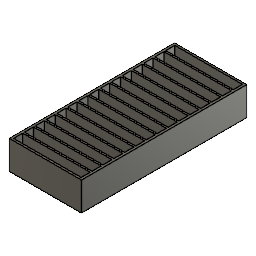
GBA Stand v4 (Autodesk Fusion 360 design; units mm, degrees)
Autodesk Fusion 360 part; units mm, degrees
sketch "Sketch1" plane through (0, 0, 0) normal (0, 1, 0) x (1, 0, 0)
  line L0 (2.75, 1.25) -> (2.75, 0)
  line L1 (2.75, 1.25) -> (54.15, 1.25)
  line L2 (54.15, 1.25) -> (54.15, 5.25)
  line L3 (54.15, 5.25) -> (2.75, 5.25)
  line L4 (2.75, 5.25) -> (2.75, 1.25)
  line L5 (0, 0) -> (56.9, 0)
  line L6 (56.9, 0) -> (56.9, 7.3)
  line L7 (56.9, 7.3) -> (0, 7.3)
  line L8 (0, 7.3) -> (0, 0)
  line L9 (-2, -2) -> (58.9, -2)
  line L10 (58.9, -2) -> (58.9, 9.3)
  line L11 (58.9, 9.3) -> (-2, 9.3)
  line L12 (-2, 9.3) -> (-2, -2)
  line L13 (58.9, -2) -> (58.9, 9.3)
  line L14 (58.9, 9.3) -> (-2, 9.3)
  line L15 (-2, 9.3) -> (-2, -2)
  line L16 (-2, -2) -> (58.9, -2)
  line L17 (2.75, 1.25) -> (54.15, 1.25)
  line L18 (2.75, 1.25) -> (2.75, 0)
  line L19 (54.15, 1.25) -> (54.15, 5.25)
  line L20 (54.15, 5.25) -> (2.75, 5.25)
  line L21 (2.75, 5.25) -> (2.75, 1.25)
  line L22 (0, 0) -> (56.9, 0)
  line L23 (56.9, 0) -> (56.9, 7.3)
  line L24 (0, 7.3) -> (0, 0)
  line L25 (56.9, 7.3) -> (0, 7.3)
  line L26 (58.9, 7.3) -> (58.9, 18.6)
  line L27 (58.9, 18.6) -> (-2, 18.6)
  line L28 (-2, 18.6) -> (-2, 7.3)
  line L29 (-2, 7.3) -> (58.9, 7.3)
  line L30 (2.75, 10.55) -> (54.15, 10.55)
  line L31 (2.75, 10.55) -> (2.75, 9.3)
  line L32 (54.15, 10.55) -> (54.15, 14.55)
  line L33 (54.15, 14.55) -> (2.75, 14.55)
  line L34 (2.75, 14.55) -> (2.75, 10.55)
  line L35 (0, 9.3) -> (56.9, 9.3)
  line L36 (56.9, 9.3) -> (56.9, 16.6)
  line L37 (0, 16.6) -> (0, 9.3)
  line L38 (56.9, 16.6) -> (0, 16.6)
  line L39 (58.9, 16.6) -> (58.9, 27.9)
  line L40 (58.9, 27.9) -> (-2, 27.9)
  line L41 (-2, 27.9) -> (-2, 16.6)
  line L42 (-2, 16.6) -> (58.9, 16.6)
  line L43 (2.75, 19.85) -> (54.15, 19.85)
  line L44 (2.75, 19.85) -> (2.75, 18.6)
  line L45 (54.15, 19.85) -> (54.15, 23.85)
  line L46 (54.15, 23.85) -> (2.75, 23.85)
  line L47 (2.75, 23.85) -> (2.75, 19.85)
  line L48 (0, 18.6) -> (56.9, 18.6)
  line L49 (56.9, 18.6) -> (56.9, 25.9)
  line L50 (0, 25.9) -> (0, 18.6)
  line L51 (56.9, 25.9) -> (0, 25.9)
  line L52 (58.9, 25.9) -> (58.9, 37.2)
  line L53 (58.9, 37.2) -> (-2, 37.2)
  line L54 (-2, 37.2) -> (-2, 25.9)
  line L55 (-2, 25.9) -> (58.9, 25.9)
  line L56 (2.75, 29.15) -> (54.15, 29.15)
  line L57 (2.75, 29.15) -> (2.75, 27.9)
  line L58 (54.15, 29.15) -> (54.15, 33.15)
  line L59 (54.15, 33.15) -> (2.75, 33.15)
  line L60 (2.75, 33.15) -> (2.75, 29.15)
  line L61 (0, 27.9) -> (56.9, 27.9)
  line L62 (56.9, 27.9) -> (56.9, 35.2)
  line L63 (0, 35.2) -> (0, 27.9)
  line L64 (56.9, 35.2) -> (0, 35.2)
  line L65 (58.9, 35.2) -> (58.9, 46.5)
  line L66 (58.9, 46.5) -> (-2, 46.5)
  line L67 (-2, 46.5) -> (-2, 35.2)
  line L68 (-2, 35.2) -> (58.9, 35.2)
  line L69 (2.75, 38.45) -> (54.15, 38.45)
  line L70 (2.75, 38.45) -> (2.75, 37.2)
  line L71 (54.15, 38.45) -> (54.15, 42.45)
  line L72 (54.15, 42.45) -> (2.75, 42.45)
  line L73 (2.75, 42.45) -> (2.75, 38.45)
  line L74 (0, 37.2) -> (56.9, 37.2)
  line L75 (56.9, 37.2) -> (56.9, 44.5)
  line L76 (0, 44.5) -> (0, 37.2)
  line L77 (56.9, 44.5) -> (0, 44.5)
  line L78 (58.9, 44.5) -> (58.9, 55.8)
  line L79 (58.9, 55.8) -> (-2, 55.8)
  line L80 (-2, 55.8) -> (-2, 44.5)
  line L81 (-2, 44.5) -> (58.9, 44.5)
  line L82 (2.75, 47.75) -> (54.15, 47.75)
  line L83 (2.75, 47.75) -> (2.75, 46.5)
  line L84 (54.15, 47.75) -> (54.15, 51.75)
  line L85 (54.15, 51.75) -> (2.75, 51.75)
  line L86 (2.75, 51.75) -> (2.75, 47.75)
  line L87 (0, 46.5) -> (56.9, 46.5)
  line L88 (56.9, 46.5) -> (56.9, 53.8)
  line L89 (0, 53.8) -> (0, 46.5)
  line L90 (56.9, 53.8) -> (0, 53.8)
  line L91 (58.9, 53.8) -> (58.9, 65.1)
  line L92 (58.9, 65.1) -> (-2, 65.1)
  line L93 (-2, 65.1) -> (-2, 53.8)
  line L94 (-2, 53.8) -> (58.9, 53.8)
  line L95 (2.75, 57.05) -> (54.15, 57.05)
  line L96 (2.75, 57.05) -> (2.75, 55.8)
  line L97 (54.15, 57.05) -> (54.15, 61.05)
  line L98 (54.15, 61.05) -> (2.75, 61.05)
  line L99 (2.75, 61.05) -> (2.75, 57.05)
  line L100 (0, 55.8) -> (56.9, 55.8)
  line L101 (56.9, 55.8) -> (56.9, 63.1)
  line L102 (0, 63.1) -> (0, 55.8)
  line L103 (56.9, 63.1) -> (0, 63.1)
  line L104 (58.9, 63.1) -> (58.9, 74.4)
  line L105 (58.9, 74.4) -> (-2, 74.4)
  line L106 (-2, 74.4) -> (-2, 63.1)
  line L107 (-2, 63.1) -> (58.9, 63.1)
  line L108 (2.75, 66.35) -> (54.15, 66.35)
  line L109 (2.75, 66.35) -> (2.75, 65.1)
  line L110 (54.15, 66.35) -> (54.15, 70.35)
  line L111 (54.15, 70.35) -> (2.75, 70.35)
  line L112 (2.75, 70.35) -> (2.75, 66.35)
  line L113 (0, 65.1) -> (56.9, 65.1)
  line L114 (56.9, 65.1) -> (56.9, 72.4)
  line L115 (0, 72.4) -> (0, 65.1)
  line L116 (56.9, 72.4) -> (0, 72.4)
  line L117 (58.9, 72.4) -> (58.9, 83.7)
  line L118 (58.9, 83.7) -> (-2, 83.7)
  line L119 (-2, 83.7) -> (-2, 72.4)
  line L120 (-2, 72.4) -> (58.9, 72.4)
  line L121 (2.75, 75.65) -> (54.15, 75.65)
  line L122 (2.75, 75.65) -> (2.75, 74.4)
  line L123 (54.15, 75.65) -> (54.15, 79.65)
  line L124 (54.15, 79.65) -> (2.75, 79.65)
  line L125 (2.75, 79.65) -> (2.75, 75.65)
  line L126 (0, 74.4) -> (56.9, 74.4)
  line L127 (56.9, 74.4) -> (56.9, 81.7)
  line L128 (0, 81.7) -> (0, 74.4)
  line L129 (56.9, 81.7) -> (0, 81.7)
  line L130 (58.9, 81.7) -> (58.9, 93)
  line L131 (58.9, 93) -> (-2, 93)
  line L132 (-2, 93) -> (-2, 81.7)
  line L133 (-2, 81.7) -> (58.9, 81.7)
  line L134 (2.75, 84.95) -> (54.15, 84.95)
  line L135 (2.75, 84.95) -> (2.75, 83.7)
  line L136 (54.15, 84.95) -> (54.15, 88.95)
  line L137 (54.15, 88.95) -> (2.75, 88.95)
  line L138 (2.75, 88.95) -> (2.75, 84.95)
  line L139 (0, 83.7) -> (56.9, 83.7)
  line L140 (56.9, 83.7) -> (56.9, 91)
  line L141 (0, 91) -> (0, 83.7)
  line L142 (56.9, 91) -> (0, 91)
  line L143 (58.9, 91) -> (58.9, 102.3)
  line L144 (58.9, 102.3) -> (-2, 102.3)
  line L145 (-2, 102.3) -> (-2, 91)
  line L146 (-2, 91) -> (58.9, 91)
  line L147 (2.75, 94.25) -> (54.15, 94.25)
  line L148 (2.75, 94.25) -> (2.75, 93)
  line L149 (54.15, 94.25) -> (54.15, 98.25)
  line L150 (54.15, 98.25) -> (2.75, 98.25)
  line L151 (2.75, 98.25) -> (2.75, 94.25)
  line L152 (0, 93) -> (56.9, 93)
  line L153 (56.9, 93) -> (56.9, 100.3)
  line L154 (0, 100.3) -> (0, 93)
  line L155 (56.9, 100.3) -> (0, 100.3)
  line L156 (58.9, 100.3) -> (58.9, 111.6)
  line L157 (58.9, 111.6) -> (-2, 111.6)
  line L158 (-2, 111.6) -> (-2, 100.3)
  line L159 (-2, 100.3) -> (58.9, 100.3)
  line L160 (2.75, 103.55) -> (54.15, 103.55)
  line L161 (2.75, 103.55) -> (2.75, 102.3)
  line L162 (54.15, 103.55) -> (54.15, 107.55)
  line L163 (54.15, 107.55) -> (2.75, 107.55)
  line L164 (2.75, 107.55) -> (2.75, 103.55)
  line L165 (0, 102.3) -> (56.9, 102.3)
  line L166 (56.9, 102.3) -> (56.9, 109.6)
  line L167 (0, 109.6) -> (0, 102.3)
  line L168 (56.9, 109.6) -> (0, 109.6)
  line L169 (58.9, 109.6) -> (58.9, 120.9)
  line L170 (58.9, 120.9) -> (-2, 120.9)
  line L171 (-2, 120.9) -> (-2, 109.6)
  line L172 (-2, 109.6) -> (58.9, 109.6)
  line L173 (2.75, 112.85) -> (54.15, 112.85)
  line L174 (2.75, 112.85) -> (2.75, 111.6)
  line L175 (54.15, 112.85) -> (54.15, 116.85)
  line L176 (54.15, 116.85) -> (2.75, 116.85)
  line L177 (2.75, 116.85) -> (2.75, 112.85)
  line L178 (0, 111.6) -> (56.9, 111.6)
  line L179 (56.9, 111.6) -> (56.9, 118.9)
  line L180 (0, 118.9) -> (0, 111.6)
  line L181 (56.9, 118.9) -> (0, 118.9)
  line L182 (58.9, 118.9) -> (58.9, 130.2)
  line L183 (58.9, 130.2) -> (-2, 130.2)
  line L184 (-2, 130.2) -> (-2, 118.9)
  line L185 (-2, 118.9) -> (58.9, 118.9)
  line L186 (2.75, 122.15) -> (54.15, 122.15)
  line L187 (2.75, 122.15) -> (2.75, 120.9)
  line L188 (54.15, 122.15) -> (54.15, 126.15)
  line L189 (54.15, 126.15) -> (2.75, 126.15)
  line L190 (2.75, 126.15) -> (2.75, 122.15)
  line L191 (0, 120.9) -> (56.9, 120.9)
  line L192 (56.9, 120.9) -> (56.9, 128.2)
  line L193 (0, 128.2) -> (0, 120.9)
  line L194 (56.9, 128.2) -> (0, 128.2)
  line L195 (58.9, 128.2) -> (58.9, 139.5)
  line L196 (58.9, 139.5) -> (-2, 139.5)
  line L197 (-2, 139.5) -> (-2, 128.2)
  line L198 (-2, 128.2) -> (58.9, 128.2)
  line L199 (2.75, 131.45) -> (54.15, 131.45)
  line L200 (2.75, 131.45) -> (2.75, 130.2)
  line L201 (54.15, 131.45) -> (54.15, 135.45)
  line L202 (54.15, 135.45) -> (2.75, 135.45)
  line L203 (2.75, 135.45) -> (2.75, 131.45)
  line L204 (0, 130.2) -> (56.9, 130.2)
  line L205 (56.9, 130.2) -> (56.9, 137.5)
  line L206 (0, 137.5) -> (0, 130.2)
  line L207 (56.9, 137.5) -> (0, 137.5)
  point P0 (0, 9.3)
  point P1 (0, 18.6)
  point P2 (0, 27.9)
  point P3 (0, 37.2)
  point P4 (0, 46.5)
  point P5 (0, 55.8)
  point P6 (0, 65.1)
  point P7 (0, 74.4)
  point P8 (0, 83.7)
  point P9 (0, 93)
  point P10 (0, 102.3)
  point P11 (0, 111.6)
  point P12 (0, 120.9)
  point P13 (0, 130.2)
  constraint horizontal L1
  constraint vertical L2
  constraint horizontal L3
  constraint vertical L4
  constraint horizontal L5
  constraint vertical L6
  constraint horizontal L7
  constraint vertical L8
  constraint coincident L5.start L8.end
  constraint horizontal L9
  constraint vertical L10
  constraint horizontal L11
  constraint vertical L12
  constraint horizontal L17
  constraint vertical L19
  constraint horizontal L20
  constraint vertical L21
  constraint horizontal L22
  constraint vertical L23
  constraint horizontal L25
  constraint vertical L24
  constraint horizontal L16
  constraint vertical L13
  constraint horizontal L14
  constraint vertical L15
  constraint horizontal L30
  constraint vertical L32
  constraint horizontal L33
  constraint vertical L34
  constraint horizontal L35
  constraint vertical L36
  constraint horizontal L38
  constraint vertical L37
  constraint coincident P0 L35.start
  constraint horizontal L29
  constraint vertical L26
  constraint horizontal L27
  constraint vertical L28
  constraint horizontal L43
  constraint vertical L45
  constraint horizontal L46
  constraint vertical L47
  constraint horizontal L48
  constraint vertical L49
  constraint horizontal L51
  constraint vertical L50
  constraint coincident P1 L48.start
  constraint horizontal L42
  constraint vertical L39
  constraint horizontal L40
  constraint vertical L41
  constraint horizontal L56
  constraint vertical L58
  constraint horizontal L59
  constraint vertical L60
  constraint horizontal L61
  constraint vertical L62
  constraint horizontal L64
  constraint vertical L63
  constraint coincident P2 L61.start
  constraint horizontal L55
  constraint vertical L52
  constraint horizontal L53
  constraint vertical L54
  constraint horizontal L69
  constraint vertical L71
  constraint horizontal L72
  constraint vertical L73
  constraint horizontal L74
  constraint vertical L75
  constraint horizontal L77
  constraint vertical L76
  constraint coincident P3 L74.start
  constraint horizontal L68
  constraint vertical L65
  constraint horizontal L66
  constraint vertical L67
  constraint horizontal L82
  constraint vertical L84
  constraint horizontal L85
  constraint vertical L86
  constraint horizontal L87
  constraint vertical L88
  constraint horizontal L90
  constraint vertical L89
  constraint coincident P4 L87.start
  constraint horizontal L81
  constraint vertical L78
  constraint horizontal L79
  constraint vertical L80
  constraint horizontal L95
  constraint vertical L97
  constraint horizontal L98
  constraint vertical L99
  constraint horizontal L100
  constraint vertical L101
  constraint horizontal L103
  constraint vertical L102
  constraint coincident P5 L100.start
  constraint horizontal L94
  constraint vertical L91
  constraint horizontal L92
  constraint vertical L93
  constraint horizontal L108
  constraint vertical L110
  constraint horizontal L111
  constraint vertical L112
  constraint horizontal L113
  constraint vertical L114
  constraint horizontal L116
  constraint vertical L115
  constraint coincident P6 L113.start
  constraint horizontal L107
  constraint vertical L104
  constraint horizontal L105
  constraint vertical L106
  constraint horizontal L121
  constraint vertical L123
  constraint horizontal L124
  constraint vertical L125
  constraint horizontal L126
  constraint vertical L127
  constraint horizontal L129
  constraint vertical L128
  constraint coincident P7 L126.start
  constraint horizontal L120
  constraint vertical L117
  constraint horizontal L118
  constraint vertical L119
  constraint horizontal L134
  constraint vertical L136
  constraint horizontal L137
  constraint vertical L138
  constraint horizontal L139
  constraint vertical L140
  constraint horizontal L142
  constraint vertical L141
  constraint coincident P8 L139.start
  constraint horizontal L133
  constraint vertical L130
  constraint horizontal L131
  constraint vertical L132
  constraint horizontal L147
  constraint vertical L149
  constraint horizontal L150
  constraint vertical L151
  constraint horizontal L152
  constraint vertical L153
  constraint horizontal L155
  constraint vertical L154
  constraint coincident P9 L152.start
  constraint horizontal L146
  constraint vertical L143
  constraint horizontal L144
  constraint vertical L145
  constraint horizontal L160
  constraint vertical L162
  constraint horizontal L163
  constraint vertical L164
  constraint horizontal L165
  constraint vertical L166
  constraint horizontal L168
  constraint vertical L167
  constraint coincident P10 L165.start
  constraint horizontal L159
  constraint vertical L156
  constraint horizontal L157
  constraint vertical L158
  constraint horizontal L173
  constraint vertical L175
  constraint horizontal L176
  constraint vertical L177
  constraint horizontal L178
  constraint vertical L179
  constraint horizontal L181
  constraint vertical L180
  constraint coincident P11 L178.start
  constraint horizontal L172
  constraint vertical L169
  constraint horizontal L170
  constraint vertical L171
  constraint horizontal L186
  constraint vertical L188
  constraint horizontal L189
  constraint vertical L190
  constraint horizontal L191
  constraint vertical L192
  constraint horizontal L194
  constraint vertical L193
  constraint coincident P12 L191.start
  constraint horizontal L185
  constraint vertical L182
  constraint horizontal L183
  constraint vertical L184
  constraint horizontal L199
  constraint vertical L201
  constraint horizontal L202
  constraint vertical L203
  constraint horizontal L204
  constraint vertical L205
  constraint horizontal L207
  constraint vertical L206
  constraint coincident P13 L204.start
  constraint horizontal L198
  constraint vertical L195
  constraint horizontal L196
  constraint vertical L197
extrude "Extrude1" add sketch "Sketch1" along normal blind 9 contours L1 L2 L3 L4 L17 L19 L20 L21 | L5 L6 L8 L9 L10 L12 L13 L15 L16 L22 L23 L24 L29 | L7 L10 L11 L12 L13 L14 L15 L25 L26 L28 L29 L35 | L11 L14 L28 L37 L42 | L11 L14 L26 L36 L42 | L26 L27 L28 L38 L39 L41 L42 L48 | L27 L41 L50 L55 | L27 L39 L49 L55 | L39 L40 L41 L51 L52 L54 L55 L61 | L40 L54 L63 L68 | L40 L52 L62 L68 | L52 L53 L54 L64 L65 L67 L68 L74 | L53 L67 L76 L81 | L53 L65 L75 L81 | L65 L66 L67 L77 L78 L80 L81 L87 | L66 L80 L89 L94 | L66 L78 L88 L94 | L78 L79 L80 L90 L91 L93 L94 L100 | L79 L93 L102 L107 | L79 L91 L101 L107 | L91 L92 L93 L103 L104 L106 L107 L113 | L92 L106 L115 L120 | L92 L104 L114 L120 | L104 L105 L106 L116 L117 L119 L120 L126 | L105 L119 L128 L133 | L105 L117 L127 L133 | L117 L118 L119 L129 L130 L132 L133 L139 | L118 L132 L141 L146 | L118 L130 L140 L146 | L130 L131 L132 L142 L143 L145 L146 L152 | L131 L145 L154 L159 | L131 L143 L153 L159 | L143 L144 L145 L155 L156 L158 L159 L165 | L144 L158 L167 L172 | L144 L156 L166 L172 | L156 L157 L158 L168 L169 L171 L172 L178 | L157 L171 L180 L185 | L157 L169 L179 L185 | L169 L170 L171 L181 L182 L184 L185 L191 | L170 L184 L193 L198 | L170 L182 L192 L198 | L182 L183 L184 L194 L195 L197 L198 L204 | L183 L195 L196 L197 L205 L206 L207 | L30 L32 L33 L34 | L43 L45 L46 L47 | L56 L58 L59 L60 | L69 L71 L72 L73 | L82 L84 L85 L86 | L95 L97 L98 L99 | L108 L110 L111 L112 | L121 L123 L124 L125 | L134 L136 L137 L138 | L147 L149 L150 L151 | L160 L162 L163 L164 | L173 L175 L176 L177 | L186 L188 L189 L190 | L199 L201 L202 L203 makes body 1 at (37.0167, 3, -5.25) makes body 2 at (37.0167, 3, -51.75) makes body 3 at (37.0167, 3, -88.95) makes body 4 at (37.0167, 3, -126.15) makes body 5 at (37.0167, 3, -116.85) makes body 6 at (37.0167, 3, -79.65) makes body 7 at (37.0167, 3, -42.45) makes body 8 at (37.0167, 3, -33.15) makes body 9 at (37.0167, 3, -14.55) makes body 10 at (37.0167, 3, -61.05) makes body 11 at (37.0167, 3, -98.25) makes body 12 at (37.0167, 3, -135.45) makes body 13 at (37.0167, 3, -107.55) makes body 14 at (37.0167, 3, -70.35) makes body 15 at (37.0167, 3, -23.85) makes body 16 at (58.2333, 0, -73.7333)
sketch "Sketch2" plane through (0, 0, 0) normal (0, 1, 0) x (1, 0, 0)
  line L0 (-2, -2) -> (58.9, -2)
  line L1 (58.9, -2) -> (58.9, 139.5)
  line L2 (58.9, 139.5) -> (-2, 139.5)
  line L3 (-2, 139.5) -> (-2, -2)
  point P0 (-2, -2)
  point P1 (58.9, 139.5)
  constraint horizontal L0
  constraint vertical L1
  constraint horizontal L2
  constraint vertical L3
  constraint coincident P1 L1.end
  constraint coincident P0 L0.start
extrude "Extrude2" add sketch "Sketch2" against normal blind 1.6 bodies 1 2 3 4 5 6 7 8 9 10 11 12 13 14 15 16
extrude "Extrude3" add 1 faces at (58.2333, 9, -83.0333) along direction (0, 1, 0) blind 14 on bodies 1 bodies 1
extrude "Extrude4" cut 15 faces at (0, 15.3333, -135.0667) (0, 15.3333, -123.3333) (0, 15.3333, -114.0333) (0, 15.3333, -104.7333) (0, 15.3333, -97.8667) (0, 15.3333, -86.1333) (0, 15.3333, -79.2667) (0, 15.3333, -69.9667) (0, 15.3333, -58.2333) (0, 15.3333, -51.3667) (0, 15.3333, -42.0667) (0, 15.3333, -30.3333) (0, 15.3333, -21.0333) (0, 7.6667, -14.1667) (0, 15.3333, -4.8667) along direction (-1, 0, 0) blind 0.5 on bodies 1 bodies 1
extrude "Extrude5" add 1 faces at (-2, 14.8, -45.1667) along direction (-1, 0, 0) blind 0.5 on bodies 1 bodies 1
extrude "Extrude6" cut 15 faces at (56.9, 15.3333, -14.1667) (56.9, 15.3333, -2.4333) (56.9, 7.6667, -21.0333) (56.9, 7.6667, -30.3333) (56.9, 7.6667, -39.6333) (56.9, 7.6667, -48.9333) (56.9, 7.6667, -58.2333) (56.9, 15.3333, -67.5333) (56.9, 15.3333, -76.8333) (56.9, 7.6667, -86.1333) (56.9, 15.3333, -95.4333) (56.9, 15.3333, -104.7333) (56.9, 7.6667, -114.0333) (56.9, 7.6667, -123.3333) (56.9, 15.3333, -132.6333) along direction (1, 0, 0) blind 0.5 on bodies 1 bodies 1
extrude "Extrude7" add 1 faces at (58.9, 14.8, -45.1667) along direction (1, 0, 0) blind 0.5 on bodies 1 bodies 1
extrude "Extrude8" cut 1 faces at (38.1, 15.3333, -130.2) along direction (0, 0, 1) blind 0.25 on bodies 1 bodies 1
extrude "Extrude9" cut 1 faces at (38.1, 15.3333, -120.9) along direction (0, 0, 1) blind 0.25 on bodies 1 bodies 1
extrude "Extrude10" cut 1 faces at (38.1, 15.3333, -111.6) along direction (0, 0, 1) blind 0.25 on bodies 1 bodies 1
extrude "Extrude11" cut 1 faces at (38.1, 15.3333, -102.3) along direction (0, 0, 1) blind 0.25 on bodies 1 bodies 1
extrude "Extrude12" cut 1 faces at (38.1, 15.3333, -93) along direction (0, 0, 1) blind 0.25 on bodies 1 bodies 1
extrude "Extrude13" cut 1 faces at (38.1, 15.3333, -83.7) along direction (0, 0, 1) blind 0.25 on bodies 1 bodies 1
extrude "Extrude14" cut 1 faces at (38.1, 15.3333, -74.4) along direction (0, 0, 1) blind 0.25 on bodies 1 bodies 1
extrude "Extrude15" cut 1 faces at (38.1, 15.3333, -65.1) along direction (0, 0, 1) blind 0.25 on bodies 1 bodies 1
extrude "Extrude16" cut 1 faces at (38.1, 15.3333, -55.8) along direction (0, 0, 1) blind 0.25 on bodies 1 bodies 1
extrude "Extrude17" cut 1 faces at (38.1, 15.3333, -46.5) along direction (0, 0, 1) blind 0.25 on bodies 1 bodies 1
extrude "Extrude18" cut 1 faces at (38.1, 15.3333, -37.2) along direction (0, 0, 1) blind 0.25 on bodies 1 bodies 1
extrude "Extrude19" cut 1 faces at (38.1, 15.3333, -27.9) along direction (0, 0, 1) blind 0.25 on bodies 1 bodies 1
extrude "Extrude20" cut 1 faces at (38.1, 15.3333, -18.6) along direction (0, 0, 1) blind 0.25 on bodies 1 bodies 1
extrude "Extrude21" cut 1 faces at (38.1, 15.3333, -9.3) along direction (0, 0, 1) blind 0.25 on bodies 1 bodies 1
extrude "Extrude22" cut 1 faces at (18.8, 7.6667, 0) along direction (0, 0, 1) blind 0.25 on bodies 1 bodies 1
extrude "Extrude23" cut 1 faces at (38.1, 7.6667, -7.3) along direction (0, 0, -1) blind 0.25 on bodies 1 bodies 1
extrude "Extrude24" cut 1 faces at (18.8, 15.3333, -16.6) along direction (0, 0, -1) blind 0.25 on bodies 1 bodies 1
extrude "Extrude25" cut 1 faces at (18.8, 15.3333, -25.9) along direction (0, 0, -1) blind 0.25 on bodies 1 bodies 1
extrude "Extrude26" cut 1 faces at (18.8, 15.3333, -35.2) along direction (0, 0, -1) blind 0.25 on bodies 1 bodies 1
extrude "Extrude27" cut 1 faces at (18.8, 15.3333, -44.5) along direction (0, 0, -1) blind 0.25 on bodies 1 bodies 1
extrude "Extrude28" cut 1 faces at (18.8, 15.3333, -53.8) along direction (0, 0, -1) blind 0.25 on bodies 1 bodies 1
extrude "Extrude29" cut 1 faces at (18.8, 15.3333, -63.1) along direction (0, 0, -1) blind 0.25 on bodies 1 bodies 1
extrude "Extrude30" cut 1 faces at (18.8, 15.3333, -72.4) along direction (0, 0, -1) blind 0.25 on bodies 1 bodies 1
extrude "Extrude31" cut 1 faces at (18.8, 15.3333, -81.7) along direction (0, 0, -1) blind 0.25 on bodies 1 bodies 1
extrude "Extrude32" cut 1 faces at (18.8, 15.3333, -91) along direction (0, 0, -1) blind 0.25 on bodies 1 bodies 1
extrude "Extrude33" cut 1 faces at (18.8, 15.3333, -100.3) along direction (0, 0, -1) blind 0.25 on bodies 1 bodies 1
extrude "Extrude34" cut 1 faces at (18.8, 15.3333, -109.6) along direction (0, 0, -1) blind 0.25 on bodies 1 bodies 1
extrude "Extrude35" cut 1 faces at (18.8, 15.3333, -118.9) along direction (0, 0, -1) blind 0.25 on bodies 1 bodies 1
extrude "Extrude36" cut 1 faces at (18.8, 15.3333, -128.2) along direction (0, 0, -1) blind 0.25 on bodies 1 bodies 1
extrude "Extrude37" cut 1 faces at (18.8, 15.3333, -137.5) along direction (0, 0, -1) blind 0.25 on bodies 1 bodies 1
extrude "Extrude38" cut 15 faces at (19.8833, 9, -3.9167) (19.8833, 9, -13.2167) (19.8833, 9, -22.5167) (19.8833, 9, -31.8167) (19.8833, 9, -41.1167) (19.8833, 9, -50.4167) (19.8833, 9, -59.7167) (19.8833, 9, -69.0167) (19.8833, 9, -78.3167) (19.8833, 9, -87.6167) (19.8833, 9, -96.9167) (19.8833, 9, -106.2167) (19.8833, 9, -115.5167) (19.8833, 9, -124.8167) (19.8833, 9, -134.1167) along direction (0, -1, 0) blind 9 on bodies 1 bodies 1
